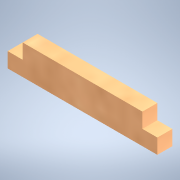
# Autodesk Inventor part: beam2
Saved by Autodesk Inventor 2022 (Build 260153000, 153)
## iProperties
Created: 2021-12-11
Part Number: beam2
Material: Wood (Cherry)
Document SubType Name: Modeling
Designer: dangl
Density: 0.63 g/cm^3
Appearance: Cherry - Natural Low Gloss
Author: dangl
Autodesk Inventor part; units mm, degrees
ref_plane "YZ Plane" through (0, 0, 0) normal (1, 0, 0) x (0, 1, 0)
ref_plane "XZ Plane" through (0, 0, 0) normal (0, 1, 0) x (-1, 0, 0)
ref_plane "XY Plane" through (0, 0, 0) normal (0, 0, 1) x (1, 0, 0)
sketch "Sketch1" plane through (0, 0, 0) normal (0, 0, 1) x (1, 0, 0)
  line L0 (-20, -4) -> (0, -4)
  line L1 (0, -4) -> (0, -2)
  line L2 (-18, 0) -> (-18, -2)
  line L3 (-18, -2) -> (-20, -2)
  line L4 (-2, 0) -> (-2, -2)
  line L5 (-2, -2) -> (0, -2)
  line L6 (-2, 0) -> (-18, 0)
  line L7 (-20, -2) -> (-20, -4)
  point P0 (0, 0)
  dimension "d0" = 4
  dimension "d1" = 20
  dimension "d2" = 2
  dimension "d3" = 2
  dimension "d4" = 2
  constraints: 16 end point, 2 parallel, 1 horizontal, 1 perpendicular, 1 point on line
  measures "d0" distance of L0.end point (0, 0)
  measures "d1" distance of L0.start L0.end
  measures "d2" distance of L2.end L3.end
  measures "d3" distance of L1.end L4.end
  measures "d4" distance of L2.start L2.end
extrude "Extrusion1" add sketch "Sketch1" along normal blind 2
body "Solid1"
